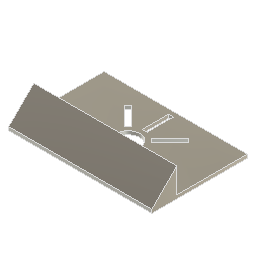
Мусорница под сверление (Autodesk Fusion 360 design; units mm, degrees)
Autodesk Fusion 360 part; units mm, degrees
note: some values were not read from the file. Chosen so that the rebuilt part matches the saved one: which face or edge a step refers to. Set by a fixed rule: which sketch regions a step uses.
sketch "Sketch1" plane through (0, 0, 0) normal (0, 0, 1) x (1, 0, 0)
  circle A0 centre (0, 0) radius 10
  line L0 (40, 40) -> (-40, 40)
  line L1 (-40, -40) -> (40, -40)
  line L2 (36, 2) -> (14, 2)
  line L3 (14, 2) -> (14, -2)
  line L4 (14, -2) -> (36, -2)
  line L5 (36, -2) -> (36, 2)
  line L6 (36, 2) -> (14, -2) construction
  line L7 (14, 2) -> (36, -2) construction
  line L8 (24.0416, 26.8701) -> (8.4853, 11.3137)
  line L9 (8.4853, 11.3137) -> (11.3137, 8.4853)
  line L10 (11.3137, 8.4853) -> (26.8701, 24.0416)
  line L11 (26.8701, 24.0416) -> (24.0416, 26.8701)
  line L12 (-2, 36) -> (-2, 14)
  line L13 (-2, 14) -> (2, 14)
  line L14 (2, 14) -> (2, 36)
  line L15 (2, 36) -> (-2, 36)
  line L16 (-26.8701, 24.0416) -> (-11.3137, 8.4853)
  line L17 (-11.3137, 8.4853) -> (-8.4853, 11.3137)
  line L18 (-8.4853, 11.3137) -> (-24.0416, 26.8701)
  line L19 (-24.0416, 26.8701) -> (-26.8701, 24.0416)
  line L20 (-36, -2) -> (-14, -2)
  line L21 (-14, -2) -> (-14, 2)
  line L22 (-14, 2) -> (-36, 2)
  line L23 (-36, 2) -> (-36, -2)
  line L24 (60, 40) -> (-60, 40)
  line L25 (-60, 40) -> (-60, -40)
  line L26 (-60, -40) -> (60, -40)
  line L27 (60, -40) -> (60, 40)
  line L28 (60, 40) -> (-60, -40) construction
  line L29 (-60, 40) -> (60, -40) construction
  point P0 (25, 0)
  dimension "d2" = 360
  constraint coincident A0.centre origin
  constraint horizontal L0
  constraint parallel L0 L1
  constraint horizontal L2
  constraint perpendicular L2 L3
  constraint parallel L2 L4
  constraint parallel L3 L5
  constraint coincident L6 P0
  constraint coincident L7 P0
  constraint horizontal L24
  constraint perpendicular L24 L25
  constraint parallel L24 L26
  constraint parallel L25 L27
  constraint coincident L28 A0.centre
  constraint coincident L29 A0.centre
extrude "Extrude1" add sketch "Sketch1" along normal blind 3
sketch "Sketch2" plane through (40, 0, 0) normal (1, 0, 0) x (0, 1, 0)
  line L0 (-40, 0) -> (40, 0)
  line L1 (40, 0) -> (40, 3)
  line L2 (40, 3) -> (-40, 3)
  line L3 (-40, 3) -> (-40, 0)
  line L4 (-40, 3) -> (-19, 24)
  line L5 (-19, 24) -> (-19, 3)
  line L6 (-38.5858, 1.5858) -> (-21, 19.1716)
  line L7 (-21, 19.1716) -> (-21, 3)
  line L8 (-21, 19.1716) -> (-19, 21.1716)
  dimension "d5" = 2
  constraint coincident L2.end L3.start
  constraint coincident L2 L5.end
  constraint perpendicular L2 L5
  constraint coincident L5 L8.end
  constraint parallel L6 L8
extrude "Extrude2" add sketch "Sketch2" along normal blind -100 and the other way blind -20 contours L2 L4 L5 L6 L8 | L2 L6 L7 | L2 L5 L7 L8
extrude "Extrude3" cut sketch "Sketch2" along normal blind -95 and the other way blind -17 contours L2 L6 L7 | L2 L5 L7 L8
